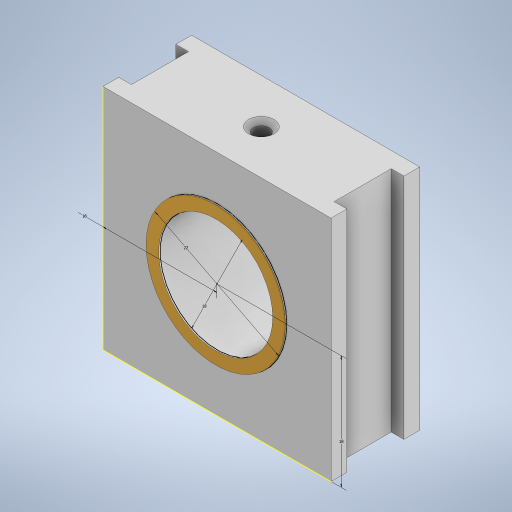
# Autodesk Inventor part: HUDSON 1-08 AXLE BLOCK
Saved by Autodesk Inventor 2024.2 (Build 282272000, 272)
## iProperties
Created: 2024-10-05
Part Number: HUDSON 1-08 AXLE BLOCK
Material: Generic
Document SubType Name: Modeling
Designer: Jimena Brenes
Density: 1 g/cm^3
Appearance: Default
Author: Jimena Brenes
Autodesk Inventor part; units mm, degrees
note: some values were not read from the file. Chosen so that the rebuilt part matches the saved one: direction of "Hole2".
ref_plane "YZ Plane" through (0, 0, 0) normal (1, 0, 0) x (0, 1, 0)
ref_plane "XZ Plane" through (0, 0, 0) normal (0, 1, 0) x (-1, 0, 0)
ref_plane "XY Plane" through (0, 0, 0) normal (0, 0, 1) x (1, 0, 0)
sketch "Sketch1" plane through (0, 0, 0) normal (0, 1, 0) x (-1, 0, 0)
  line L0 (0, 0) -> (-36, 0)
  line L1 (-36, -14) -> (0, -14)
  line L2 (0, 0) -> (0, -2.5)
  line L3 (-2, -2.5) -> (-2, -11.5)
  line L4 (-34, -2.5) -> (-34, -11.5)
  line L5 (0.1666, -2.5) -> (-2, -2.5)
  line L6 (0, -14) -> (0, -11.5)
  line L7 (0, -11.5) -> (-2, -11.5)
  line L8 (-34, -11.5) -> (-36, -11.5)
  line L9 (-36, -11.5) -> (-36, -14)
  line L10 (-34, -2.5) -> (-36, -2.5)
  line L11 (-36, -2.5) -> (-36, 0)
  dimension "d1" = 14
  dimension "d2" = 36
  dimension "d3" = 2.5
  dimension "d4" = 9
  dimension "d5" = 9
  dimension "d6" = 32
  dimension "d8" = 9
  dimension "d9" = 36
  constraints: 24 end point, 4 perpendicular, 4 vertical, 2 horizontal, 1 parallel, 1 point on line
  measures "d1" distance of L0.end L1.start
  measures "d2" distance of L1.start L1.end
  measures "d3" distance of L0.start L2.end
  measures "d4" distance of L3.start L3.end
  measures "d5" distance of L4.start L4.end
  measures "d6" distance between parallel lines of L4 L3
  measures "d8" distance from line of L3.end L5
  measures "d9" distance of L0.start L0.end
extrude "Extrusion1" add sketch "Sketch1" along normal blind 36
sketch "Sketch2" plane through (0, 36, 0) normal (0, 1, 0) x (1, 0, 0)
  circle A0 centre (18, 7) radius 1.25
  line L0 (34, 2.5) -> (34, 11.5) projected
  line L1 (0, 0) -> (36, 0) projected
  dimension "d12" = 2.5
  dimension "d13" = 16
  dimension "d14" = 7
  constraints: 1 centre point
  measures "d12" diameter of A0
  measures "d13" distance from line of L0 A0.centre
  measures "d14" distance from line of L1 A0.centre
sketch "Sketch3" plane through (0, 0, 0) normal (0, 0, 1) x (1, 0, 0)
  circle A0 centre (18, 18) radius 11
  circle A1 centre (18, 18) radius 9
  line L0 (0, 0) -> (36, 0) projected
  line L1 (0, 0) -> (0, 36) projected
  dimension "d15" = 22
  dimension "d16" = 18
  dimension "d17" = 18
  dimension "d18" = 18
  constraints: 2 centre point, 1 coincident
  measures "d15" diameter of A0
  measures "d16" diameter of A1
  measures "d17" distance from line of L0 A0.centre
  measures "d18" distance from line of L1 A0.centre
hole "Hole1" at (18, 18, 0) direction (0, 0, -1) diameter 18 end through all
extrude "Extrusion2" add sketch "Sketch3" along normal blind 0.2
hole "Hole2" at (18, 36, -7) direction (0, -1, 0) diameter 2.5 end up to surface countersink diameter 4 countersink angle 90
body "Solid1"
